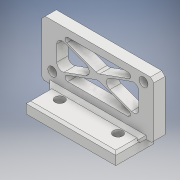
# Autodesk Inventor part: Ping-front
Saved by Autodesk Inventor 2018.3 (Build 223284000, 284)
## iProperties
Created: 2018-12-18
Part Number: Ping-front
Material: ABS プラスチック
Document SubType Name: Modeling
Designer: shun2
Density: 1.06 g/cm^3
Appearance: 滑らか - 白
Author: shun2
Autodesk Inventor part; units mm, degrees
ref_plane "YZ Plane" through (0, 0, 0) normal (1, 0, 0) x (0, 1, 0)
ref_plane "XZ Plane" through (0, 0, 0) normal (0, 1, 0) x (-1, 0, 0)
ref_plane "XY Plane" through (0, 0, 0) normal (0, 0, 1) x (1, 0, 0)
sketch "スケッチ1" plane through (0, 0, 0) normal (0, 0, 1) x (1, 0, 0)
  line L0 (0, 0) -> (40, 0)
  line L1 (40, 0) -> (40, 17)
  line L2 (40, 17) -> (0, 17)
  line L3 (0, 17) -> (0, 0)
  circle A0 centre (7, 8) radius 2.1
  circle A1 centre (33, 8) radius 2.1
  dimension "d0" = 40
  dimension "d1" = 17
  dimension "d2" = 4.2
  dimension "d3" = 4.2
  constraints: 8 end point, 2 centre point, 2 parallel, 1 horizontal, 1 perpendicular
  measures "d0" distance of L2.end L1.end
  measures "d1" distance of L1.end L0.end
  measures "d2" diameter of A0
  measures "d3" diameter of A1
extrude "押し出し1" add sketch "スケッチ1" along normal blind 5 contours L3 L2 L1 L0 | A0 | A1
sketch "スケッチ2" plane through (0, 0, 0) normal (0, 0, -1) x (-1, 0, 0)
  line L0 (0, 0) -> (-40, 0) projected
  line L1 (0, 17) -> (0, 0) projected
  line L2 (-40, 17) -> (0, 17) projected
  line L3 (-40, 0) -> (-40, 17) projected
  circle A0 centre (-7, 8) radius 2.1 projected
  circle A1 centre (-33, 8) radius 2.1 projected
extrude "押し出し2" cut sketch "スケッチ2" against normal blind 5 contours A0 | A1
sketch "スケッチ3" plane through (0, 0, 5) normal (0, 0, 1) x (1, 0, 0)
  line L0 (-5, 17) -> (45, 17)
  line L1 (45, 17) -> (45, 12)
  line L2 (45, 12) -> (-5, 12)
  line L3 (-5, 12) -> (-5, 17)
  point P0 (0, 0)
  dimension "d8" = 50
  dimension "d9" = 5
  constraints: 8 end point, 2 parallel, 1 horizontal, 1 perpendicular
  measures "d8" distance of L1.end L2.end
  measures "d9" distance of L0.end L1.end
extrude "押し出し3" add sketch "スケッチ3" along normal blind 25
sketch "スケッチ4" plane through (40, 12, 5) normal (0, -1, 0) x (1, 0, 0)
  line L0 (2.903, 24.0436) -> (-42.797, 24.0436)
  line L1 (-42.797, 24.0436) -> (-42.797, 2.7436)
  line L2 (-42.797, 2.7436) -> (2.903, 2.7436)
  line L3 (2.903, 2.7436) -> (2.903, 24.0436)
  circle A0 centre (0.403, 21.5436) radius 1.55
  circle A1 centre (-40.297, 5.2436) radius 1.55
  circle A2 centre (-7.747, 13.3936) radius 8.15
  circle A3 centre (-32.147, 13.3936) radius 8.15
  line L4 (0, 0) -> (-40, 0) projected
  circle A4 centre (0.403, 21.5436) radius 2
  circle A5 centre (-40.297, 5.2436) radius 2
  point P0 (-40, -5)
  point P1 (-19.947, 10.8936)
  dimension "d12" = 4
  dimension "d13" = 4
  constraints: 8 end point, 6 centre point, 2 coincident, 2 equal radius, 2 perpendicular, 1 parallel
  measures "d12" diameter of A4
  measures "d13" diameter of A5
extrude "押し出し4" cut sketch "スケッチ4" against normal blind 5 contours A0 | A1 | A4 | A5
chamfer "面取り1" distance 1.5 angle 45 3 edges at (-5, 14.5, 30) (45, 14.5, 30) (20, 12, 5)
chamfer "面取り2" distance 1.5 angle 45 2 edges at (0, 14.5, 5) (40, 14.5, 5)
chamfer "面取り3" distance 1.5 angle 45 4 edges at (0, 12, 4.25) (0, 12, 5.75) (40, 12, 4.25) (40, 12, 5.75)
chamfer "面取り4" distance 1 angle 45 5 edges at (-5, 14.5, 5) (45, 14.5, 5) (0, 5.25, 5) (20, 0, 5) (40, 5.25, 5)
sketch "スケッチ5" plane through (-3.5, 12, 30) normal (0, -1, 0) x (1, 0, 0)
  line L0 (0, 0) -> (47, 0) projected
  line L1 (23.5, 0) -> (23.5, -19.0027)
  line L2 (-1.5, -24) -> (-1.5, -1.5) projected
  line L3 (-1.5, -12.75) -> (3.191, -12.75)
  line L4 (18.0971, -9.4165) -> (8.3932, -5.8846)
  line L5 (24.2624, -11.6605) -> (34.589, -11.6605) construction
  line L6 (18.0971, -13.9044) -> (8.3932, -17.4364)
  line L7 (24.2624, -11.6605) -> (34.589, -11.6605) construction
  line L8 (5.1885, -15.1924) -> (5.1885, -8.1286)
  arc A0 (18.0971, -13.9044) -> (18.0971, -9.4165) centre (17.2803, -11.6605) ccw
  arc A1 (8.3932, -5.8846) -> (5.1885, -8.1286) centre (7.5765, -8.1286) ccw
  arc A2 (5.1885, -15.1924) -> (8.3932, -17.4364) centre (7.5765, -15.1924) ccw
  line L9 (28.9029, -9.4165) -> (38.6068, -5.8846)
  line L10 (28.9029, -13.9044) -> (38.6068, -17.4364)
  line L11 (41.8115, -15.1924) -> (41.8115, -8.1286)
  arc A3 (28.9029, -9.4165) -> (28.9029, -13.9044) centre (29.7197, -11.6605) ccw
  arc A4 (41.8115, -8.1286) -> (38.6068, -5.8846) centre (39.4235, -8.1286) ccw
  arc A5 (38.6068, -17.4364) -> (41.8115, -15.1924) centre (39.4235, -15.1924) ccw
  line L12 (24.3167, -10.1619) -> (37.3327, -5.4245)
  line L13 (23.5, -10.4592) -> (37.3513, -10.4592) construction
  line L14 (22.6833, -10.1619) -> (9.6673, -5.4245)
  line L15 (23.5, -10.4592) -> (37.3513, -10.4592) construction
  line L16 (10.0756, -3.1085) -> (36.9244, -3.1085)
  arc A6 (22.6833, -10.1619) -> (24.3167, -10.1619) centre (23.5, -7.9179) ccw
  arc A7 (10.0756, -3.1085) -> (9.6673, -5.4245) centre (10.0756, -4.3025) ccw
  arc A8 (37.3327, -5.4245) -> (36.9244, -3.1085) centre (36.9244, -4.3025) ccw
  line L17 (24.3167, -13.159) -> (37.3327, -17.8965)
  line L18 (23.5, -12.8618) -> (37.3513, -12.8618) construction
  line L19 (22.6833, -13.159) -> (9.6673, -17.8965)
  line L20 (10.0756, -20.2125) -> (36.9244, -20.2125)
  arc A9 (24.3167, -13.159) -> (22.6833, -13.159) centre (23.5, -15.403) ccw
  arc A10 (9.6673, -17.8965) -> (10.0756, -20.2125) centre (10.0756, -19.0185) ccw
  arc A11 (36.9244, -20.2125) -> (37.3327, -17.8965) centre (36.9244, -19.0185) ccw
  point P0 (3.5, -30)
  point P1 (5.1885, -4.7181)
  point P2 (5.1885, -18.6028)
  point P3 (41.8115, -4.7181)
  point P4 (41.8115, -18.6028)
  point P5 (43.6959, -3.1085)
  point P6 (3.3041, -3.1085)
  point P7 (37.3513, -12.8618)
  point P8 (23.5, -11.6605)
  dimension "d28" = 20.298
  dimension "d29" = 160
  dimension "d30" = 20.298
  dimension "d31" = 160
  dimension "d32" = 2.388
  dimension "d33" = 21.492
  dimension "d34" = 20
  dimension "d35" = 21.492
  dimension "d36" = 160
  dimension "d37" = 2.388
  dimension "d38" = 1.194
  constraints: 38 end point, 24 point on circle, 19 point on line, 12 centre point, 12 tangent, 5 horizontal, 4 equal length, 3 equal radius, 2 midpoint, 1 vertical
  measures "d28" distance of L5.start point (5.188, -4.718)
  measures "d29" angle of L5 L4
  measures "d30" distance of L5.start point (5.188, -18.603)
  measures "d31" angle of L6 L7
  measures "d32" radius of A0
  measures "d33" distance of L13.start point (43.696, -3.108)
  measures "d34" angle of L13 L12
  measures "d35" distance of L13.start point (3.304, -3.108)
  measures "d36" angle of L15 L14
  measures "d37" radius of A6
  measures "d38" radius of A7
extrude "押し出し5" cut sketch "スケッチ5" against normal blind 5
